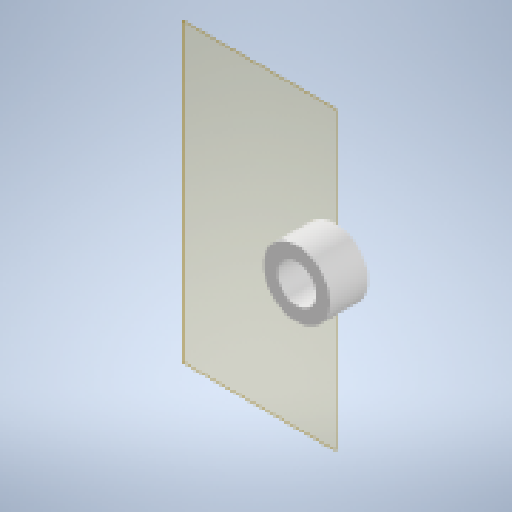
# Autodesk Inventor part: belt_tentioner_washer
Saved by Autodesk Inventor 2024 (Build 280153000, 153)
## iProperties
Created: 2026-02-05
Part Number: belt_tentioner_washer
Material: Generic
Document SubType Name: Modeling
Designer: SEMEN
Density: 1 g/cm^3
Appearance: Default
Author: SEMEN
Autodesk Inventor part; units mm, degrees
ref_plane "YZ Plane" through (0, 0, 0) normal (1, 0, 0) x (0, 1, 0)
ref_plane "XZ Plane" through (0, 0, 0) normal (0, 1, 0) x (-1, 0, 0)
ref_plane "XY Plane" through (0, 0, 0) normal (0, 0, 1) x (1, 0, 0)
ref_plane "Work Plane1" through (154.2208, -12.0981, 0.5428) normal (0, 0, 1) x (1, 0, 0)
sketch "Sketch1" plane through (154.2208, -12.0981, 0.5428) normal (0, 0, 1) x (1, 0, 0)
  circle A0 centre (10.8766, 2.2345) radius 2.75 projected
  circle A1 centre (10.8766, 2.2345) radius 4.75
  point P0 (-154.2208, 12.0981)
  dimension "d0" = 2
  constraints: 1 centre point
  measures "d0" radial gap between concentric circles of A0 A1
ref_plane "Work Plane2" through (156.0974, -18.8636, -1.7364) normal (0, 0, -1) x (0, 1, 0)
ref_plane "Work Plane3" through (156.0974, -18.8636, 6.0428) normal (0, 0, -1) x (0, 1, 0)
extrude "Extrusion1" add sketch "Sketch1" along normal up to surface (5.5 mm away)
body "Solid1"
